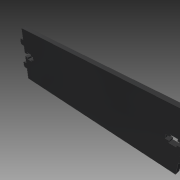
# Autodesk Inventor part: front_panel_2004_bottom
Saved by Autodesk Inventor 2014 (Build 180170000, 170)
## iProperties
Created: 2014-01-11
Part Number: front_panel_2004_bottom
Material: Generic
Document SubType Name: Modeling
Designer: buben
Density: 1 g/cm^3
Appearance: Anodized - Dark Gray
Author: buben
Autodesk Inventor part; units mm, degrees
ref_plane "YZ Plane" through (0, 0, 0) normal (1, 0, 0) x (0, 1, 0)
ref_plane "XZ Plane" through (0, 0, 0) normal (0, 1, 0) x (-1, 0, 0)
ref_plane "XY Plane" through (0, 0, 0) normal (0, 0, 1) x (1, 0, 0)
sketch "Sketch1" plane through (0, 0, 0) normal (0, 1, 0) x (-1, 0, 0)
  line L0 (0, 0) -> (220, 0)
  line L1 (220, 0) -> (220, 70)
  line L2 (220, 70) -> (0, 70)
  line L3 (0, 70) -> (0, 0)
  dimension "d11" = 220
  dimension "d16" = 70
  constraints: 8 end point, 2 parallel, 1 horizontal, 1 perpendicular
  measures "d11" distance of L0.start L0.end
  measures "d16" distance of L2.end L0.start
extrude "Extrusion3" add sketch "Sketch1" along normal blind 6
sketch "Sketch5" plane through (0, 0, 0) normal (0, -1, 0) x (1, 0, 0)
  line L0 (0, 0) -> (-220, 0) projected
  line L1 (0, 70) -> (0, 0) projected
  line L2 (-220, 70) -> (0, 70) projected
  line L3 (-220, 0) -> (-220, 70) projected
  line L4 (-220, 55) -> (-224, 55)
  line L5 (-226, 53) -> (-226, 49)
  line L6 (-224, 47) -> (-220, 47)
  line L7 (-220, 47) -> (-220, 55)
  line L8 (-220, 23) -> (-224, 23)
  line L9 (-226, 21) -> (-226, 17)
  line L10 (-224, 15) -> (-220, 15)
  line L11 (-220, 15) -> (-220, 23)
  line L12 (0, 55) -> (4, 55)
  line L13 (6, 53) -> (6, 49)
  line L14 (4, 47) -> (0, 47)
  line L15 (0, 47) -> (0, 55)
  line L16 (0, 23) -> (4, 23)
  line L17 (6, 21) -> (6, 17)
  line L18 (4, 15) -> (0, 15)
  line L19 (0, 15) -> (0, 23)
  arc A0 (-224, 55) -> (-226, 53) centre (-224, 53) ccw
  arc A1 (-226, 49) -> (-224, 47) centre (-224, 49) ccw
  arc A2 (-224, 23) -> (-226, 21) centre (-224, 21) ccw
  arc A3 (-226, 17) -> (-224, 15) centre (-224, 17) ccw
  arc A4 (4, 47) -> (6, 49) centre (4, 49) ccw
  arc A5 (6, 53) -> (4, 55) centre (4, 53) ccw
  arc A6 (6, 21) -> (4, 23) centre (4, 21) ccw
  arc A7 (4, 15) -> (6, 17) centre (4, 17) ccw
  dimension "d61" = 2
  dimension "d62" = 8
  dimension "d63" = 8
  dimension "d64" = 6
  dimension "d65" = 15
  dimension "d66" = 15
  dimension "d67" = 6
  constraints: 32 end point, 16 point on circle, 16 tangent, 8 centre point, 8 parallel, 7 equal radius, 6 collinear, 4 horizontal, 4 perpendicular, 4 point on line
  measures "d61" radius of A0
  measures "d62" distance between parallel lines of L6 L4
  measures "d63" distance between parallel lines of L10 L8
  measures "d64" distance between parallel lines of L3 L5
  measures "d65" distance between parallel lines of L2 L4
  measures "d66" distance between parallel lines of L0 L10
  measures "d67" distance between parallel lines of L1 L13
extrude "Extrusion6" add sketch "Sketch5" against normal blind 6 contours L1 L16 A6 L17 A7 L18 | L10 A3 L9 A2 L8 L3 | L1 L12 A5 L13 A4 L14 | L6 A1 L5 A0 L4 L3
sketch "Sketch6" plane through (0, 0, 0) normal (0, -1, 0) x (1, 0, 0)
  line L0 (0, 0) -> (-220, 0) projected
  line L1 (-220, 70) -> (0, 70) projected
  line L2 (-220, 23) -> (-220, 47) projected
  line L3 (-110, 70) -> (-110, 0) construction
  line L4 (-203.7, 37.25) -> (-203.7, 32.75)
  line L5 (-220, 32.75) -> (-220, 37.25)
  line L6 (-215, 39.75) -> (-207.7, 39.75)
  line L7 (-207.7, 30.25) -> (-215, 30.25)
  line L8 (-220, 37.25) -> (-215, 37.25)
  line L9 (-207.7, 37.25) -> (-203.7, 37.25)
  line L10 (-203.7, 32.75) -> (-207.7, 32.75)
  line L11 (-215, 32.75) -> (-220, 32.75)
  line L12 (-215, 30.25) -> (-215, 32.75)
  line L13 (-215, 37.25) -> (-215, 39.75)
  line L14 (-207.7, 39.75) -> (-207.7, 37.25)
  line L15 (-207.7, 32.75) -> (-207.7, 30.25)
  line L16 (-16.3, 37.25) -> (-16.3, 32.75)
  line L17 (0, 32.75) -> (0, 37.25)
  line L18 (-5, 39.75) -> (-12.3, 39.75)
  line L19 (-12.3, 30.25) -> (-5, 30.25)
  line L20 (0, 37.25) -> (-5, 37.25)
  line L21 (-12.3, 37.25) -> (-16.3, 37.25)
  line L22 (-16.3, 32.75) -> (-12.3, 32.75)
  line L23 (-5, 32.75) -> (0, 32.75)
  line L24 (-5, 30.25) -> (-5, 32.75)
  line L25 (-5, 37.25) -> (-5, 39.75)
  line L26 (-12.3, 39.75) -> (-12.3, 37.25)
  line L27 (-12.3, 32.75) -> (-12.3, 30.25)
  point P0 (-220, 35)
  point P1 (0, 35)
  dimension "d70" = 2.5
  dimension "d71" = 2.5
  dimension "d72" = 4.5
  dimension "d73" = 5
  dimension "d74" = 7.3
  dimension "d75" = 4
  constraints: 50 end point, 13 symmetric about line, 10 parallel, 4 collinear, 4 midpoint, 4 perpendicular, 3 horizontal
  measures "d70" distance of L10.end L7.start
  measures "d71" distance of L6.end L9.start
  measures "d72" distance of L4.start L4.end
  measures "d73" distance of L11.start L5.start
  measures "d74" distance of L7.start L7.end
  measures "d75" distance of L4.end L10.end
extrude "Extrusion7" cut sketch "Sketch6" against normal blind 6
equation "\"d66\" = d65"
equation "\"d71\" = d70"
body "Solid2"
